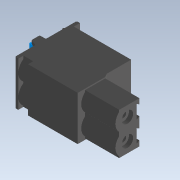
# Autodesk Inventor part: 5065608 2GD-1RR5,08-CLP-CBL
Saved by Autodesk Inventor 2021 (Build 250183000, 183)
## iProperties
Part Number: 5065608 2GD-1RR5,08-CLP-CBL
Material: Generic
Catalog Web Link: www.cadenas.de
Description: NEKM-C6 (p)-Terminal strip
Vendor: FESTO
Document SubType Name: Modeling
Designer: partserver
Manufacturer: FESTO
Mass: 2.55188 g
Surface Area: 17.4369 cm^2
Volume: 2.55188 cm^3
Density: 1 g/cm^3
Appearance: PSOLRGB-80-80-80
Categories: <MemberInstance><Categories><Category DisplayName="" Mnemonic="CABLEANDHARNESS" InternalName="e4a7e005-5e42-4d16-b293-125e7f0d0512"><Category DisplayName="" Mnemonic="CONNECTORS" InternalName="6f634eba-a678-4820-a31d-2c2d5ee6728e"><CategoryParameter DisplayName="" Mnemonic="REFDES" InternalName="c3740e8c-60ab-4d5d-8584-52b73222f2f0"/><Category DisplayName="" Mnemonic="DISCRETEWIRE" InternalName="9a3407de-09b2-4cdb-8c40-9708d5144a28"/></Category></Category></Categories><FamilyTemplate><FamilyTemplateParameters></FamilyTemplateParameters></FamilyTemplate><CategoryParameterMap><ParamToTemplateMap><ParamToTemplate CategoryParameter="//CategoryParameter[@InternalName='c3740e8c-60ab-4d5d-8584-52b73222f2f0']" ConstantValue=""/></ParamToTemplateMap></CategoryParameterMap></MemberInstance>
Category: PARTsolutions
Company: FESTO
PSOL_IDENT_0: {$CADENAS_DATA\23d-libs\festo\parts\n\nekm\parts\nekm_c6_parts.prj},200 {VTYP=3D},{NB=5065608 2GD-1R
PSOL_IDENT_1: R5,08-CLP-CBL},{LINA=5065608 2GD-1RR5,08-CLP-CBL},{NN=NEKM-C6 (p)},{DATE=16.05.2019 05:36:58},{GEOMD
PSOL_IDENT_2: ATE=16.05.2019 05:36:56},{VERSION=},{LINEID=110},{WBVAR=},{WBNUMERIC=}  {NB=5065608 2GD-1RR5,08-CLP-
PSOL_IDENT_3: CBL},{LINA=5065608 2GD-1RR5,08-CLP-CBL},{KT=DUMMY},{TNR=5065608},{TYP=2GD-1RR5,08-CLP-CBL},{VERS=2},
PSOL_IDENT_4: {N=2},{L=10.780},{L1=2.850}
NB: 5065608 2GD-1RR5,08-CLP-CBL
NN: NEKM-C6 (p)
NT: Terminal strip
NBSYN: $TNR. $TYP.
LINA: 5065608 2GD-1RR5,08-CLP-CBL
CATALOG: Festo
TNR: 5065608
TYP: 2GD-1RR5,08-CLP-CBL
VERS: 2
N: 2
L: 10.78
L1: 2.85
SUPPLIER: FESTO
ARTICLENO: 5065608 2GD-1RR5,08-CLP-CBL
BOMINFO: 5065608 2GD-1RR5,08-CLP-CBL
CREATOR: CADENAS GmbH
Title: 5065608 2GD-1RR5,08-CLP-CBL
Author: Cadenas PARTsolutions
Comments: Terminal strip
Autodesk Inventor part; units mm, degrees
sketch "Sketch_1" plane through (0, 0, 0) normal (0, 0, 1) x (1, 0, 0)
  line L0 (0, 6) -> (0, -7.5)
  line L1 (0, -7.5) -> (14.43, -7.5)
  arc A0 (14.43, -7.5) -> (14.73, -7.2) centre (14.43, -7.2) ccw
  line L2 (14.73, -7.2) -> (14.73, 4.1)
  arc A1 (14.73, 4.1) -> (14.73, 4.5) centre (14.73, 4.3) ccw
  line L3 (14.73, 4.5) -> (14.73, 7.2)
  arc A2 (14.73, 7.2) -> (14.43, 7.5) centre (14.43, 7.2) ccw
  line L4 (14.43, 7.5) -> (13.93, 7.5)
  line L5 (13.93, 7.5) -> (13.93, 6)
  line L6 (13.93, 6) -> (0, 6)
  constraints: 14 end point, 6 point on circle, 3 centre point
extrude "Extrusion1" add sketch "Sketch_1" along normal mid plane 10.78
sketch "Sketch_2" plane through (0, 0, 5.39) normal (0, 0, 1) x (1, 0, 0)
  line L0 (14.73, 0.2) -> (14.73, -2.756)
  arc A0 (14.9274, -2.4741) -> (14.73, -2.756) centre (15.03, -2.756) ccw
  line L1 (14.9274, -2.4741) -> (16.0326, -2.0718)
  arc A1 (16.0326, -2.0718) -> (16.23, -1.7899) centre (15.93, -1.7899) ccw
  line L2 (16.23, -1.7899) -> (16.23, -0.3)
  arc A2 (16.23, -0.3) -> (15.93, 0) centre (15.93, -0.3) ccw
  line L3 (15.93, 0) -> (14.93, 0)
  arc A3 (14.73, 0.2) -> (14.93, 0) centre (14.93, 0.2) ccw
  constraints: 8 end point, 8 point on circle, 4 centre point
extrude "Extrusion2" add sketch "Sketch_2" against normal blind 0.8
pattern_linear "Rectangular Pattern1" count 2 spacing 9.98 along (0, 0, -1) of "Extrusion2"
sketch "Sketch_40" plane through (0, 0, 0.49) normal (0, 0, 1) x (1, 0, 0)
  line L0 (14.73, 0.2) -> (14.73, -2.756)
  arc A0 (14.9274, -2.4741) -> (14.73, -2.756) centre (15.03, -2.756) ccw
  line L1 (14.9274, -2.4741) -> (16.0326, -2.0718)
  arc A1 (16.0326, -2.0718) -> (16.23, -1.7899) centre (15.93, -1.7899) ccw
  line L2 (16.23, -1.7899) -> (16.23, -0.3)
  arc A2 (16.23, -0.3) -> (15.93, 0) centre (15.93, -0.3) ccw
  line L3 (15.93, 0) -> (14.93, 0)
  arc A3 (14.73, 0.2) -> (14.93, 0) centre (14.93, 0.2) ccw
  constraints: 8 end point, 8 point on circle, 4 centre point
extrude "Extrusion3" add sketch "Sketch_40" against normal blind 0.98
sketch "Sketch_6" plane through (0, 0, 4.49) normal (0, 0, 1) x (1, 0, 0)
  line L0 (14.73, -2.075) -> (16.6, -2.075)
  arc A0 (16.6, -2.075) -> (16.8, -1.875) centre (16.6, -1.875) ccw
  line L1 (16.8, -1.875) -> (16.8, -1.7601)
  arc A1 (16.8, -1.7601) -> (16.6041, -1.516) centre (16.55, -1.7601) ccw
  line L2 (16.6041, -1.516) -> (15.9359, -1.3679)
  arc A2 (15.9359, -0.7821) -> (15.9359, -1.3679) centre (16.0008, -1.075) ccw
  line L3 (15.9359, -0.7821) -> (16.6041, -0.634)
  arc A3 (16.6041, -0.634) -> (16.8, -0.3899) centre (16.55, -0.3899) ccw
  line L4 (16.8, -0.3899) -> (16.8, -0.275)
  arc A4 (16.8, -0.275) -> (16.6, -0.075) centre (16.6, -0.275) ccw
  line L5 (16.6, -0.075) -> (14.73, -0.075)
  line L6 (14.73, -0.075) -> (14.73, -2.075)
  constraints: 14 end point, 10 point on circle, 5 centre point
extrude "Extrusion4" add sketch "Sketch_6" against normal blind 3.9
pattern_linear "Rectangular Pattern2" count 2 spacing 5.08 along (0, 0, -1) of "Extrusion4"
sketch "Sketch_8" plane through (0, -4.65, 0) normal (0, 1, 0) x (1, 0, 0)
  line L0 (14.73, -2.74) -> (11.73, -2.74)
  line L1 (11.73, -2.74) -> (11.73, -0.74)
  line L2 (11.73, -0.74) -> (14.53, -0.74)
  arc A0 (14.53, -0.74) -> (14.73, -0.54) centre (14.53, -0.54) ccw
  line L3 (14.73, -0.54) -> (14.73, -2.74)
  line L4 (14.73, -2.74) -> (11.73, -2.74)
  constraints: 10 end point, 2 point on circle, 1 centre point
revolve "Revolution1" cut sketch "Sketch_8" angle 360 about axis through (14.73, -4.65, 2.74) along (1, 0, 0)
pattern_linear "Rectangular Pattern3" count 2 spacing 5.08 along (0, 0, -1) of "Revolution1"
sketch "Sketch_10" plane through (13.93, 0, 0) normal (1, 0, 0) x (0, 0, -1)
  line L0 (-4.8313, 6) -> (-0.2487, 6)
  arc A0 (-0.2487, 6) -> (-4.8313, 6) centre (-2.54, 5) ccw
  constraints: 2 end point, 2 point on circle, 1 centre point
extrude "Extrusion5" add sketch "Sketch_10" against normal blind 9.7
pattern_linear "Rectangular Pattern4" count 2 spacing 5.08 along (0, 0, -1) of "Extrusion5"
sketch "Sketch_12" plane through (0, 0, 0) normal (0, 0, 1) x (1, 0, 0)
  line L0 (2, 7.5) -> (2, 6)
  line L1 (2, 6) -> (4.23, 6)
  line L2 (4.23, 6) -> (5.73, 7.5)
  line L3 (5.73, 7.5) -> (2, 7.5)
  constraints: 8 end point
extrude "Extrusion6" cut sketch "Sketch_12" along normal mid plane 10.78
sketch "Sketch_13" plane through (14.73, 0, 0) normal (1, 0, 0) x (0, 0, -1)
  line L0 (-3.715, 5.775) -> (-3.715, 4.6)
  line L1 (-3.715, 4.6) -> (-1.365, 4.6)
  line L2 (-1.365, 4.6) -> (-1.365, 5.775)
  arc A0 (-1.365, 5.775) -> (-3.715, 5.775) centre (-2.54, 5.775) ccw
  constraints: 6 end point, 2 point on circle, 1 centre point
extrude "Extrusion7" cut sketch "Sketch_13" against normal blind 9.325
pattern_linear "Rectangular Pattern5" count 2 spacing 5.08 along (0, 0, -1) of "Extrusion7"
sketch "Sketch_15" plane through (0, 7.5, 0) normal (0, 1, 0) x (1, 0, 0)
  arc A0 (5.405, -1.365) -> (5.405, -3.715) centre (5.405, -2.54) ccw
  line L0 (5.405, -3.715) -> (6.58, -3.715)
  line L1 (6.58, -3.715) -> (6.58, -1.365)
  line L2 (6.58, -1.365) -> (5.405, -1.365)
  constraints: 6 end point, 2 point on circle, 1 centre point
extrude "Extrusion8" cut sketch "Sketch_15" against normal blind 2.9
pattern_linear "Rectangular Pattern6" count 2 spacing 5.08 along (0, 0, -1) of "Extrusion8"
sketch "Sketch_17" plane through (3.13, 0, 0) normal (1, 0, 0) x (0, 0, -1)
  line L0 (-2.54, 6) -> (-2.54, 6.3)
  arc A0 (-2.09, 6) -> (-2.54, 6.3) centre (-2.5483, 5.8001) ccw
  line L1 (-2.09, 6) -> (-2.54, 6)
  line L2 (-2.54, 6) -> (-2.54, 6.3)
  constraints: 6 end point, 2 point on circle, 1 centre point
revolve "Revolution2" add sketch "Sketch_17" angle 360 about axis through (3.13, 6, 2.54) along (0, -1, 0)
pattern_linear "Rectangular Pattern7" count 2 spacing 5.08 along (0, 0, -1) of "Revolution2"
sketch "Sketch_25" plane through (0, 0, 0) normal (0, 0, 1) x (1, 0, 0)
  line L0 (-0.5, -0.795) -> (-0.5, -7.5)
  line L1 (-0.5, -7.5) -> (0, -7.5)
  line L2 (0, -7.5) -> (0, 0.071)
  line L3 (0, 0.071) -> (-0.5, -0.795)
  constraints: 8 end point
extrude "Extrusion9" add sketch "Sketch_25" along normal mid plane 10.78
sketch "Sketch_35" plane through (-0.5, 0, 0) normal (1, 0, 0) x (0, 0, -1)
  line L0 (-5.08, -5.71) -> (-4.6607, -5.71)
  arc A0 (-4.6607, -5.71) -> (-0.4193, -5.71) centre (-2.54, -3.71) ccw
  line L1 (-0.4193, -5.71) -> (0.4193, -5.71)
  arc A1 (0.4193, -5.71) -> (4.6607, -5.71) centre (2.54, -3.71) ccw
  line L2 (4.6607, -5.71) -> (5.08, -5.71)
  line L3 (5.08, -5.71) -> (5.08, -0.795)
  line L4 (5.08, -0.795) -> (3.797, -0.795)
  line L5 (3.797, -0.795) -> (4.1896, -1.475)
  line L6 (4.1896, -1.475) -> (0.8934, -1.475)
  line L7 (0.8934, -1.475) -> (1.286, -0.795)
  line L8 (1.286, -0.795) -> (-1.283, -0.795)
  line L9 (-1.283, -0.795) -> (-0.8904, -1.475)
  line L10 (-0.8904, -1.475) -> (-4.1866, -1.475)
  line L11 (-4.1866, -1.475) -> (-3.794, -0.795)
  line L12 (-3.794, -0.795) -> (-5.08, -0.795)
  line L13 (-5.08, -0.795) -> (-5.08, -5.71)
  constraints: 28 end point, 4 point on circle, 2 centre point
extrude "Extrusion10" add sketch "Sketch_35" against normal blind 8.3
sketch "Sketch13" plane through (-8.8, 0, 0) normal (-1, 0, 0) x (0, 0, 1)
  point P0 (2.54, -3.71)
hole "Hole1" at (-8.8, -3.71, 2.54) direction (1, 0, 0) diameter 1.4 depth 2 counterbore diameter 2.8 counterbore depth 1
pattern_linear "Rectangular Pattern8" count 2 spacing 5.08 along (0, 0, -1) of "Hole1"
sketch "Sketch_30" plane through (0, 0, 2.54) normal (0, 0, 1) x (1, 0, 0)
  arc A0 (-4.9014, 1.2616) -> (-4.86, 0.947) centre (-4.76, 1.1202) ccw
  line L0 (-4.86, 0.947) -> (-4.1642, 0.5453)
  arc A1 (-4.1642, 0.5453) -> (-3.8021, 0.5929) centre (-4.0142, 0.8051) ccw
  line L1 (-3.8021, 0.5929) -> (-3.53, 0.865)
  line L2 (-3.53, 0.865) -> (-0.3256, 1.0049)
  arc A2 (-0.3, 0.406) -> (-0.3256, 1.0049) centre (-0.3, 0.706) ccw
  arc A3 (-0.3, 0.406) -> (-0.5, 0.206) centre (-0.3, 0.206) ccw
  line L3 (-0.5, 0.206) -> (-0.5, -1)
  line L4 (-0.5, -1) -> (0.5, -1)
  line L5 (0.5, -1) -> (0.5, 3.3534)
  line L6 (0.5, 3.3534) -> (0, 3.3534)
  arc A4 (-0.2325, 3.0611) -> (0, 3.3534) centre (-0.3, 3.3534) ccw
  line L7 (-0.2325, 3.0611) -> (-3.7536, 2.2482)
  arc A5 (-3.7536, 2.2482) -> (-4.1152, 2.0478) centre (-3.5849, 1.5174) ccw
  line L8 (-4.1152, 2.0478) -> (-4.9014, 1.2616)
  constraints: 18 end point, 12 point on circle, 6 centre point
extrude "Extrusion11" add sketch "Sketch_30" against normal blind 1.6
sketch "Sketch_27" plane through (11.58, 0, 0) normal (1, 0, 0) x (0, 0, -1)
  line L0 (-5.39, -8.25) -> (5.39, -8.25)
  line L1 (5.39, -8.25) -> (5.39, -6.25)
  line L2 (5.39, -6.25) -> (4.6985, -6.25)
  arc A0 (-0.0185, -6.25) -> (4.6985, -6.25) centre (2.34, -4.65) ccw
  line L3 (-0.0185, -6.25) -> (-0.3815, -6.25)
  arc A1 (-5.0985, -6.25) -> (-0.3815, -6.25) centre (-2.74, -4.65) ccw
  line L4 (-5.0985, -6.25) -> (-5.39, -6.25)
  line L5 (-5.39, -6.25) -> (-5.39, -8.25)
  constraints: 12 end point, 4 point on circle, 2 centre point
extrude "Extrusion12" cut sketch "Sketch_27" along normal blind 2.35
ref_plane "ANBAU_XY" through (0, 0, 0) normal (0, 1, 0) x (1, 0, 0)
ref_plane "ANBAU_YZ" through (0, 0, 0) normal (1, 0, 0) x (0, 0, -1)
ref_plane "ANBAU_ZX" through (0, 0, 0) normal (0, 0, -1) x (0, 1, 0)
ref_plane "CP1_XY" through (-0.5, -3.71, 0) normal (1, 0, 0) x (0, 0, -1)
ref_plane "CP1_YZ" through (-0.5, -3.71, 0) normal (0, 0, -1) x (0, 1, 0)
ref_plane "CP1_ZX" through (-0.5, -3.71, 0) normal (0, 1, 0) x (1, 0, 0)
sketch "Sketch16" plane through (14.73, 4.1, 5.39) normal (1, 0, 0) x (0, 0, -1)
  circle A0 centre (2.65, -8.75) radius 2.2 projected
sketch "Sketch17" plane through (14.73, 4.1, 5.39) normal (1, 0, 0) x (0, 0, -1)
  circle A0 centre (7.73, -8.75) radius 2.2 projected
body "Solid1"
